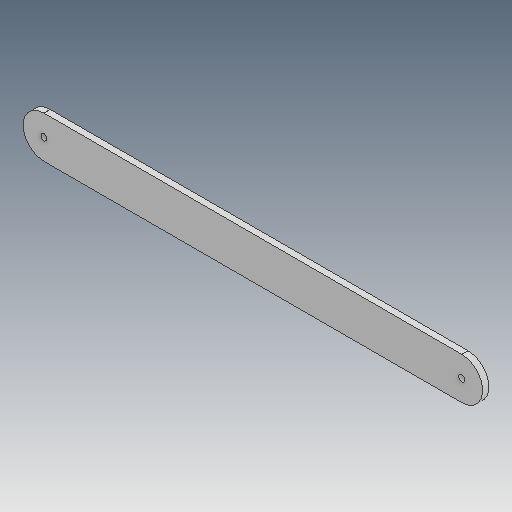
# Autodesk Inventor part: Träger vorne unten
Saved by Autodesk Inventor 2020 (Build 240168000, 168)
## iProperties
Created: 2021-06-29
Part Number: Träger vorne unten
Material: Generisch
Document SubType Name: Modeling
Designer: Mike
Density: 1 g/cm^3
Appearance: Vorgabe
Author: Mike
Autodesk Inventor part; units mm, degrees
ref_plane "YZ Plane" through (0, 0, 0) normal (1, 0, 0) x (0, 1, 0)
ref_plane "XZ Plane" through (0, 0, 0) normal (0, 1, 0) x (-1, 0, 0)
ref_plane "XY Plane" through (0, 0, 0) normal (0, 0, 1) x (1, 0, 0)
sketch "Skizze1" plane through (0, 0, 0) normal (0, 0, 1) x (1, 0, 0)
  line L0 (-221.2928, 0) -> (86.7072, 0) projected
  line L1 (0, -13.0671) -> (0, 14.9771) projected
  line L2 (-167.2928, 10.9392) -> (32.7072, 10.9392)
  line L3 (32.7072, -9.0608) -> (-167.2928, -9.0608)
  arc A0 (-167.2928, 10.9708) -> (-167.2928, -9.0292) centre (-167.2928, 0.9708) ccw
  line L4 (-167.2928, -9.0608) -> (-167.2928, -9.0292)
  line L5 (-167.2928, 10.9708) -> (-167.2928, 10.9392)
  arc A1 (32.7072, -9.0608) -> (32.7072, 10.9392) centre (32.7072, 0.9392) ccw
  point P0 (0, 0)
  point P1 (32.7072, 10.9392)
  dimension "d3" = 10
  dimension "d5" = 10
  dimension "d6" = 20
  dimension "d7" = 200
  constraints: 8 end point, 4 point on circle, 2 centre point, 1 horizontal, 1 parallel
  measures "d3" radius of A0
  measures "d5" radius of A1
  measures "d6" distance between parallel lines of L3 L2
  measures "d7" distance of A0.centre A1.centre
extrude "Extrusion1" add sketch "Skizze1" along normal blind 3
sketch "Skizze2" plane through (0, 0, 3) normal (0, 0, 1) x (1, 0, 0)
  arc A0 (32.7072, -9.0608) -> (32.7072, 10.9392) centre (32.7072, 0.9392) ccw projected
  arc A1 (-167.2928, 10.9708) -> (-167.2928, -9.0292) centre (-167.2928, 0.9708) ccw projected
  point P0 (0, 0)
  dimension "d10" = 0
  dimension "d11" = 0
  dimension "d12" = 0
  dimension "d13" = 0
  measures "d10" distance of A0.centre point (32.707, 0.939)
  measures "d11" distance of A0.centre point (32.707, 0.939)
  measures "d12" distance of A1.centre point (-167.293, 0.971)
  measures "d13" distance of A1.centre point (-167.293, 0.971)
hole "Bohrung1" at (-167.2928, 0.9708, 3) at (32.7072, 0.9392, 3) direction (0, 0, -1) diameter 3 depth 57.1 tip angle 118
